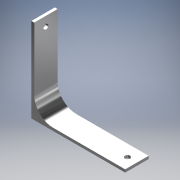
# Autodesk Inventor part: Custom Bracket
Saved by Autodesk Inventor 2019.4 (Build 234330000, 330)
## iProperties
Created: 2020-01-11
Part Number: Custom Bracket
Material: Aluminum 6061
Document SubType Name: Modeling
Designer: Mark
Mass: 28.35 g
Surface Area: 79.9 cm^2
Volume: 10.5 cm^3
Density: 2.7 g/cm^3
Appearance: Aluminum - Flat
Author: Mark
Autodesk Inventor part; units mm, degrees
ref_plane "YZ Plane" through (0, 0, 0) normal (1, 0, 0) x (0, 1, 0)
ref_plane "XZ Plane" through (0, 0, 0) normal (0, 1, 0) x (-1, 0, 0)
ref_plane "XY Plane" through (0, 0, 0) normal (0, 0, 1) x (1, 0, 0)
sketch "Sketch1" plane through (0, 0, 0) normal (0, 0, 1) x (1, 0, 0)
  line L0 (0, 0) -> (97, 0)
  line L1 (97, 0) -> (97, 3)
  line L2 (97, 3) -> (0, 3)
  line L3 (0, 3) -> (0, 0)
  line L4 (0, 0) -> (-3, 0)
  line L5 (-3, 0) -> (-3, 90)
  line L6 (-3, 90) -> (0, 90)
  line L7 (0, 90) -> (0, 0)
  dimension "d0" = 97
  dimension "d1" = 3
  dimension "d2" = 3
  dimension "d3" = 90
  constraints: 16 end point, 4 parallel, 2 horizontal, 2 perpendicular
  measures "d0" distance of L2.end L1.end
  measures "d1" distance of L0.end L1.end
  measures "d2" distance of L5.end L6.end
  measures "d3" distance of L4.end L5.end
extrude "Extrusion1" add sketch "Sketch1" along normal blind 25
sketch "Sketch2" plane through (-3, 0, 0) normal (-1, 0, 0) x (0, 0, 1)
  circle A0 centre (12.5, 80) radius 2.75
  line L0 (25, 90) -> (25, 0) projected
  line L1 (0, 90) -> (25, 90) projected
  point P0 (0, 0)
  dimension "d6" = 5.5
  dimension "d7" = 12.5
  dimension "d8" = 10
  constraints: 1 centre point
  measures "d6" diameter of A0
  measures "d7" distance from line of L0 A0.centre
  measures "d8" distance from line of L1 A0.centre
extrude "Extrusion2" cut sketch "Sketch2" against normal blind 25
sketch "Sketch3" plane through (-3, 0, 0) normal (0, -1, 0) x (1, 0, 0)
  circle A0 centre (90, 12.5) radius 2.75
  line L0 (100, 0) -> (100, 25) projected
  line L1 (0, 25) -> (100, 25) projected
  point P0 (3, 0)
  dimension "d11" = 5.5
  dimension "d12" = 10
  dimension "d13" = 12.5
  constraints: 1 centre point
  measures "d11" diameter of A0
  measures "d12" distance from line of L0 A0.centre
  measures "d13" distance from line of L1 A0.centre
extrude "Extrusion3" cut sketch "Sketch3" against normal blind 25
fillet "Fillet1" radius 20 1 edges at (0, 3, 12.5)
body "Solid1"
